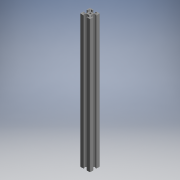
# Autodesk Inventor part: HFS5-2020-270
Saved by Autodesk Inventor 2017.3 (Build 213256000, 256)
## iProperties
Part Number: HFS5-2020-270
Material: Generic
Catalog Web Link: www.cadenas.de
Description: NFS5-2020, NFSB5-2020, HFS5-2020, HFSB5-2020, CAF5-2020, HFSY5-2020, NFSF5-2020, HFSF5-2020, HFSFB5-2020, NFST5-2020, HFST5-2020, HFSTB5-2020, HFSH5-2020, HFSC5-2020-HFS5 Series Aluminum Extrusions 20 Square -1 Slot-
Vendor: MISUMI
Document SubType Name: Modeling
Designer: partserver
Manufacturer: MISUMI
Mass: 49.1762 g
Surface Area: 472.843 cm^2
Volume: 49.1762 cm^3
Density: 1 g/cm^3
Appearance: PSOLRGB-175-175-175
Category: PARTsolutions
Company: MISUMI
Title: HFS5-2020-270
Author: Cadenas PARTsolutions
Comments: HFS5 Series Aluminum Extrusions 20 Square -1 Slot-
PSOL_IDENT_0: {$CADENAS_DATA\23d-libs\misumi\metric\38_al_extrusions_blackets\5\hfs5_2020.prj},677 {VTYP=3D},{NB=H
PSOL_IDENT_1: FS5-2020-270},{LINA=HFS5-2020-270},{NN=NFS5-2020, NFSB5-2020, HFS5-2020, HFSB5-2020, CAF5-2020, HFSY
PSOL_IDENT_2: 5-2020, NFSF5-2020, HFSF5-2020, HFSFB5-2020, NFST5-2020, HFST5-2020, HFSTB5-2020, HFSH5-2020, HFSC5-
PSOL_IDENT_3: 2020},{DATE=09.09.2019 15:28:27},{GEOMDATE=18.06.2019 07:59:14},{VERSION=},{LINEID=150},{WBVAR=L,ALT
PSOL_IDENT_4: 1,ALT2,ALT4,ALT5,CP5,DL5,DR5,ALT6,ALT9,ALT10,ALT11,HP6,NHL6,DL6,NHR6,DR6,ALT7,ALT8,NH9,AH,BH,CH,DH,E
PSOL_IDENT_5: H,NH10,AV,BV,CV,DV,EV,NH11,AP,BP,CP,DP,EP,ALT12,ALT13,Z,NH12,XA,XB,XC,XD,XE,NH13,YA,YB,YC,YD,YE,ALT1
PSOL_IDENT_6: 6,HP16,DL16,DR16,ALT17,HQ17,JLP,ALT20},{WBNUMERIC=L,NH9,AH,BH,CH,DH,EH,NH10,AV,BV,CV,DV,EV,NH11,AP,B
PSOL_IDENT_7: P,CP,DP,EP,NH12,XA,XB,XC,XD,XE,NH13,YA,YB,YC,YD,YE,HQ17,JLP}  {NB=HFS5-2020-270},{LINA=HFS5-2020-270
PSOL_IDENT_8: },{KT=DUMMY},{PN=HFS5-2020-270},{TPS=HFS5-2020},{MAT=A6N01SS-T5 Aluminum Alloy or 6005A-T5 Aluminum
PSOL_IDENT_9: Alloy},{ST=Clear Anodize},{FRMW=20},{FRMH=20},{FRD=4.2},{L=270},{MASS=0.5},{SA=183},{LX=0.742x10^4},
PSOL_IDENT_10: {LY=0.742x10^4},{ALT1=},{M1=0},{DPL1=0},{DPR1=0},{ALT1PN=},{ALT2=},{ALT2ALG= '','w/o End Tapping (He
PSOL_IDENT_11: li-Coil Insert)','LHP','with LHP (Tapping on the Left (Heli-Coil Insert))','RHP','with RHP (Tapping
PSOL_IDENT_12: on the Right (Heli-Coil Insert))','HPW','with HPW (Tapping on Both Ends (Heli-Coil Insert))' },{M2=0
PSOL_IDENT_13: },{DP2=0},{ALT2PN=},{ALT4=},{ALT4ALG= '', 'w/o SC (High Precision Cut)', 'SC', 'with SC (High Precis
PSOL_IDENT_14: ion Cut)' },{ALT4PN=},{ALT5=},{ALT5ALG= '','w/o 45 Degree Cut','1','with 45 Degree Cut' },{CP5=},{CP
PSOL_IDENT_15: 5ALG= '','N/A' },{DL5=},{DL5ALG= '','N/A' },{DR5=},{DR5ALG= '','N/A' },{FRMLALT5=0},{FRMRALT5=0},{AL
PSOL_IDENT_16: T5PN=},{ALT6=},{ALT6ALG= '','w/o Fastening Location Wrench Access Hole Alterations','1','with Fasten
PSOL_IDENT_17: ing Location Wrench Access Hole Alterations' },{ALT9=},{ALT9ALG= '','w/o Location Specified Wrench A
PSOL_IDENT_18: ccess Hole Alteratons (Horizontal)','1','with Location Specified Wrench Access Hole Alteratons (Hori
PSOL_IDENT_19: zontal)' },{ALT10=},{ALT10ALG= '','w/o Location Specified Wrench Access Hole Alteratons (Vertical)','
PSOL_IDENT_20: 1','with Location Specified Wrench Access Hole Alteratons (Vertical)' },{ALT11=},{ALT11ALG= '','w/o
PSOL_IDENT_21: Location Specified Wrench Access Hole Alteratons (Crisscross)','1','with Location Specified Wrench A
PSOL_IDENT_22: ccess Hole Alteratons (Crisscross)' },{HP6=},{HP6ALG= '','N/A' },{NHL6=},{NHL6ALG= '','N/A' },{DL6=}
PSOL_IDENT_23: ,{DL6ALG= '','N/A' },{NHR6=},{NHR6ALG= '','N/A' },{DR6=},{DR6ALG= '','N/A' },{HL6=0.000},{HL6D=0},{H
PSOL_IDENT_24: R6=0.000},{HR6D=0},{J6=0},{J6D=0},{K6=0},{K6D=0},{DD6=0.00},{DD6ALG=0},{ALT7=},{ALT7ALG= '','N/A' },
PSOL_IDENT_25: {ALT8=},{ALT8ALG= '','N/A' },{ALT678PN=},{NH9=0},{NH9MAX=5},{NH9ALG=[0]},{AH=0.0},{AHMIN=7},{AHMAX=2
PSOL_IDENT_26: 65},{AHALG=[0]},{BH=0.0},{BHMIN=2},{BHMAX=267},{BHALG=[0]},{CH=0.0},{CHMIN=2},{CHMAX=269},{CHALG=[0]
PSOL_IDENT_27: },{DH=0.0},{DHMIN=2},{DHMAX=271},{DHALG=[0]},{EH=0.0},{EHMIN=2},{EHMAX=263},{EHALG=[0]},{NH10=0},{NH
PSOL_IDENT_28: 10MAX=5},{NH10ALG=[0]},{AV=0.0},{AVMIN=7},{AVMAX=265},{AVALG=[0]},{BV=0.0},{BVMIN=2},{BVMAX=267},{BV
PSOL_IDENT_29: ALG=[0]},{CV=0.0},{CVMIN=2},{CVMAX=269},{CVALG=[0]},{DV=0.0},{DVMIN=2},{DVMAX=271},{DVALG=[0]},{EV=0
PSOL_IDENT_30: .0},{EVMIN=2},{EVMAX=263},{EVALG=[0]},{NH11=0},{NH11MAX=5},{NH11ALG=[0]},{AP=0.0},{APMIN=7},{APMAX=2
PSOL_IDENT_31: 65},{APALG=[0]},{BP=0.0},{BPMIN=2},{BPMAX=267},{BPALG=[0]},{CP=0.0},{CPMIN=2},{CPMAX=269},{CPALG=[0]
PSOL_IDENT_32: },{DP=0.0},{DPMIN=2},{DPMAX=271},{DPALG=[0]},{EP=0.0},{EPMIN=2},{EPMAX=263},{EPALG=[0]},{ALT9PN=},{A
PSOL_IDENT_33: LT10PN=},{ALT11PN=},{ALT91011PN=},{ALT12=},{ALT12ALG= '','w/o Counterbore Hole in Specified Position
PSOL_IDENT_34: (Vertical)','1','with Counterbore Hole in Specified Position (Vertical)' },{ALT13=},{ALT13ALG= '','
PSOL_IDENT_35: w/o Counterbore Hole in Specified Position (Horizontal)','1','with Counterbore Hole in Specified Pos
PSOL_IDENT_36: ition (Horizontal)' },{Z=},{ZALG= '','N/A' },{DD12=0.0},{DD112=0.0},{NH12=0},{NH12MAX=5},{NH12ALG=[0
PSOL_IDENT_37: ]},{XA=0.0},{XAMIN=7},{XAMAX=265},{XAALG=[0]},{XB=0.0},{XBMIN=2},{XBMAX=267},{XBALG=[0]},{XC=0.0},{X
PSOL_IDENT_38: CMIN=2},{XCMAX=269},{XCALG=[0]},{XD=0.0},{XDMIN=2},{XDMAX=271},{XDALG=[0]},{XE=0.0},{XEMIN=2},{XEMAX=
PSOL_IDENT_39: 263},{XEALG=[0]},{NH13=0},{NH13MAX=5},{NH13ALG=[0]},{YA=0.0},{YAMIN=7},{YAMAX=265},{YAALG=[0]},{YB=0
PSOL_IDENT_40: .0},{YBMIN=2},{YBMAX=267},{YBALG=[0]},{YC=0.0},{YCMIN=2},{YCMAX=269},{YCALG=[0]},{YD=0.0},{YDMIN=2},
PSOL_IDENT_41: {YDMAX=271},{YDALG=[0]},{YE=0.0},{YEMIN=2},{YEMAX=263},{YEALG=[0]},{ALT12PN=},{ALT13PN=},{ALT1213PN=
PSOL_IDENT_42: },{ALT16=},{ALT16ALG= '','w/o M Type Hole Alteration','1','with M Type Hole Alteration' },{HP16=},{H
PSOL_IDENT_43: P16ALG= '','N/A' },{DL16=},{DL16ALG= '','N/A' },{DR16=},{DR16ALG= '','N/A' },{H116=0},{D16=0.0},{ALT
PSOL_IDENT_44: 16PN=},{ALT17=},{ALT17ALG= '','w/o L Type Hole Alteration (Top)','1','with L Type Hole Alteration (T
PSOL_IDENT_45: op)' },{HQ17=0},{HQ17ALG=0},{JLP=0},{JLPMIN=4.9},{JLPMAX=0},{JLPALG=[0]},{L17=0},{D17=0.0},{ALT17PN=
PSOL_IDENT_46: },{ALT20=},{ALT20PN=},{ERRORALT01=OK},{ERRORALT02=OK},{ERRORALT05=OK},{ERRORALT06091=OK},{ERRORALT06
PSOL_IDENT_47: 092=OK},{ERRORALT06093=OK},{ERRORALT06094=OK},{ERRORALT06101=OK},{ERRORALT06102=OK},{ERRORALT06103=O
PSOL_IDENT_48: K},{ERRORALT06104=OK},{ERRORALT06111=OK},{ERRORALT06112=OK},{ERRORALT06113=OK},{ERRORALT06114=OK},{E
PSOL_IDENT_49: RRORALT06121=OK},{ERRORALT06122=OK},{ERRORALT06123=OK},{ERRORALT06124=OK},{ERRORALT06131=OK},{ERRORA
PSOL_IDENT_50: LT06132=OK},{ERRORALT06133=OK},{ERRORALT06134=OK},{ERRORALT0616=OK},{ERRORALT06171=OK},{ERRORALT0617
PSOL_IDENT_51: 2=OK},{ERRORALT06173=OK},{ERRORALT0911=OK},{ERRORALT0913=OK},{ERRORALT0916=OK},{ERRORALT0917=OK},{ER
PSOL_IDENT_52: RORALT1011=OK},{ERRORALT1012=OK},{ERRORALT1016=OK},{ERRORALT1017=OK},{ERRORALT1112=OK},{ERRORALT1113=
PSOL_IDENT_53: OK},{ERRORALT1116=OK},{ERRORALT1117=OK},{ERRORALT1216=OK},{ERRORALT1217=OK},{ERRORALT1316=OK},{ERROR
PSOL_IDENT_54: ALT1317=OK},{ERRORALT1617=OK},{ERRORPN=},{TFW=0}
NB: HFS5-2020-270
NN: NFS5-2020, NFSB5-2020, HFS5-2020, HFSB5-2020, CAF5-2020, HFSY5-2020, NFSF5-2020, HFSF5-2020, HFSFB5-2020, NFST5-2020, HFST5-2020, HFSTB5-2020, HFSH5-2020, HFSC5-2020
NT: HFS5 Series Aluminum Extrusions 20 Square -1 Slot-
NBSYN: $PN.
LINA: HFS5-2020-270
CATALOG: Misumi
PN: HFS5-2020-270
TPS: HFS5-2020
MAT: A6N01SS-T5 Aluminum Alloy or 6005A-T5 Aluminum Alloy
ST: Clear Anodize
L: 270
MASS: 0.5
SA: 183
LX: 0.742x10^4
LY: 0.742x10^4
ALT1: w/o End Tapping
M1: 0
DPL1: 0
DPR1: 0
ALT2: w/o End Tapping (Heli-Coil Insert)
M2: 0
DP2: 0
ALT4: w/o SC (High Precision Cut)
ALT5: w/o 45 Degree Cut
CP5: N/A
DL5: N/A
DR5: N/A
ALT6: w/o Fastening Location Wrench Access Hole Alterations
ALT9: w/o Location Specified Wrench Access Hole Alteratons (Horizontal)
ALT10: w/o Location Specified Wrench Access Hole Alteratons (Vertical)
ALT11: w/o Location Specified Wrench Access Hole Alteratons (Crisscross)
HP6: N/A
NHL6: N/A
DL6: N/A
NHR6: N/A
DR6: N/A
HL6D: 0
HR6D: 0
J6D: 0
K6D: 0
DD6: 0
ALT7: N/A
ALT8: N/A
NH9: 0
AH: 0
BH: 0
CH: 0
DH: 0
EH: 0
NH10: 0
AV: 0
BV: 0
CV: 0
DV: 0
EV: 0
NH11: 0
AP: 0
BP: 0
CP: 0
DP: 0
EP: 0
ALT12: w/o Counterbore Hole in Specified Position (Vertical)
ALT13: w/o Counterbore Hole in Specified Position (Horizontal)
Z: N/A
DD12: 0
DD112: 0
NH12: 0
XA: 0
XB: 0
XC: 0
XD: 0
XE: 0
NH13: 0
YA: 0
YB: 0
YC: 0
YD: 0
YE: 0
ALT16: w/o M Type Hole Alteration
HP16: N/A
DL16: N/A
DR16: N/A
H116: 0
D16: 0
ALT17: w/o L Type Hole Alteration (Top)
HQ17: 0
JLP: 0
D17: 0
ALT20: w/o CW (End Face C Chamfering)
SUPPLIER: MISUMI
ARTICLENO: HFS5-2020-270
BOMINFO: HFS5-2020-270
CREATOR: CADENAS GmbH
Autodesk Inventor part; units mm, degrees
ref_plane "YZ Plane" through (0, 0, 0) normal (1, 0, 0) x (0, 1, 0)
ref_plane "XZ Plane" through (0, 0, 0) normal (0, 1, 0) x (-1, 0, 0)
ref_plane "XY Plane" through (0, 0, 0) normal (0, 0, 1) x (1, 0, 0)
sketch "Sketch_1" plane through (0, 0, 0) normal (0, 0, 1) x (1, 0, 0)
  line L0 (-10, -3) -> (-10, -9)
  arc A0 (-10, -9) -> (-9, -10) centre (-9, -9) ccw
  line L1 (-9, -10) -> (-3, -10)
  line L2 (-3, -10) -> (-3, -8)
  line L3 (-3, -8) -> (-6, -8)
  line L4 (-6, -8) -> (-6, -7.0607)
  line L5 (-6, -7.0607) -> (-2.9393, -4)
  line L6 (-2.9393, -4) -> (-0.5196, -4)
  line L7 (-0.5196, -4) -> (0, -3.7)
  line L8 (0, -3.7) -> (0.5196, -4)
  line L9 (0.5196, -4) -> (2.9393, -4)
  line L10 (2.9393, -4) -> (6, -7.0607)
  line L11 (6, -7.0607) -> (6, -8)
  line L12 (6, -8) -> (3, -8)
  line L13 (3, -8) -> (3, -10)
  line L14 (3, -10) -> (9, -10)
  arc A1 (9, -10) -> (10, -9) centre (9, -9) ccw
  line L15 (10, -9) -> (10, -3)
  line L16 (10, -3) -> (8, -3)
  line L17 (8, -3) -> (8, -6)
  line L18 (8, -6) -> (7.0607, -6)
  line L19 (7.0607, -6) -> (4, -2.9393)
  line L20 (4, -2.9393) -> (4, -0.5196)
  line L21 (4, -0.5196) -> (3.7, 0)
  line L22 (3.7, 0) -> (4, 0.5196)
  line L23 (4, 0.5196) -> (4, 2.9393)
  line L24 (4, 2.9393) -> (7.0607, 6)
  line L25 (7.0607, 6) -> (8, 6)
  line L26 (8, 6) -> (8, 3)
  line L27 (8, 3) -> (10, 3)
  line L28 (10, 3) -> (10, 9)
  arc A2 (10, 9) -> (9, 10) centre (9, 9) ccw
  line L29 (9, 10) -> (3, 10)
  line L30 (3, 10) -> (3, 8)
  line L31 (3, 8) -> (6, 8)
  line L32 (6, 8) -> (6, 7.0607)
  line L33 (6, 7.0607) -> (2.9393, 4)
  line L34 (2.9393, 4) -> (0.5196, 4)
  line L35 (0.5196, 4) -> (0, 3.7)
  line L36 (0, 3.7) -> (-0.5196, 4)
  line L37 (-0.5196, 4) -> (-2.9393, 4)
  line L38 (-2.9393, 4) -> (-6, 7.0607)
  line L39 (-6, 7.0607) -> (-6, 8)
  line L40 (-6, 8) -> (-3, 8)
  line L41 (-3, 8) -> (-3, 10)
  line L42 (-3, 10) -> (-9, 10)
  arc A3 (-9, 10) -> (-10, 9) centre (-9, 9) ccw
  line L43 (-10, 9) -> (-10, 3)
  line L44 (-10, 3) -> (-8, 3)
  line L45 (-8, 3) -> (-8, 6)
  line L46 (-8, 6) -> (-7.0607, 6)
  line L47 (-7.0607, 6) -> (-4, 2.9393)
  line L48 (-4, 2.9393) -> (-4, 0.5196)
  line L49 (-4, 0.5196) -> (-3.7, 0)
  line L50 (-3.7, 0) -> (-4, -0.5196)
  line L51 (-4, -0.5196) -> (-4, -2.9393)
  line L52 (-4, -2.9393) -> (-7.0607, -6)
  line L53 (-7.0607, -6) -> (-8, -6)
  line L54 (-8, -6) -> (-8, -3)
  line L55 (-8, -3) -> (-10, -3)
  constraints: 112 end point, 8 point on circle, 4 centre point
extrude "Extrusion1" add sketch "Sketch_1" against normal blind 270
sketch "Sketch2" plane through (0, 0, -270) normal (0, 0, -1) x (-1, 0, 0)
  point P0 (0, 0)
hole "Hole1" at (0, 0, -270) direction (0, 0, 1) diameter 4.2 depth 270
ref_plane "C1_XY" through (0, 0, 0) normal (0, 0, 1) x (1, 0, 0)
ref_plane "C1_YZ" through (0, 0, 0) normal (1, 0, 0) x (0, 1, 0)
ref_plane "C1_ZX" through (0, 0, 0) normal (0, 1, 0) x (0, 0, 1)
body "Solid1"
